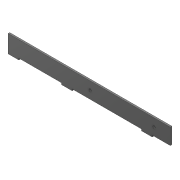
# Autodesk Inventor part: Divisória-30cm c rolamento
Saved by Autodesk Inventor 2020 (Build 240168000, 168)
## iProperties
Created: 2021-09-21
Part Number: Divisória-30cm c rolamento
Material: Generic
Document SubType Name: Modeling
Designer: pablo
Density: 1 g/cm^3
Appearance: Smooth - Black
Author: pablo
Autodesk Inventor part; units mm, degrees
ref_plane "YZ Plane" through (0, 0, 0) normal (1, 0, 0) x (0, 1, 0)
ref_plane "XZ Plane" through (0, 0, 0) normal (0, 1, 0) x (-1, 0, 0)
ref_plane "XY Plane" through (0, 0, 0) normal (0, 0, 1) x (1, 0, 0)
sketch "Sketch1" plane through (0, 0, 0) normal (0, 0, 1) x (1, 0, 0)
  line L0 (-152, 15) -> (152, 15)
  line L1 (152, 15) -> (152, -15)
  line L2 (152, -15) -> (-152, -15)
  line L3 (-152, -15) -> (-152, 15)
  line L4 (-152, 15) -> (152, -15) construction
  line L5 (152, 15) -> (-152, -15) construction
  point P0 (0, 0)
  dimension "d0" = 304
  dimension "d1" = 30
  constraints: 12 end point, 2 midpoint, 2 parallel, 1 horizontal, 1 perpendicular
  measures "d0" distance of L1.end L2.end
  measures "d1" distance of L0.end L1.end
extrude "Base" add sketch "Sketch1" along normal blind 3
sketch "Sketch2" plane through (0, 0, 3) normal (0, 0, 1) x (1, 0, 0)
  line L0 (-152, -15) -> (152, -15) projected
  line L1 (-152, -15) -> (-132, -15)
  line L2 (-132, -15) -> (-132, -18)
  line L3 (-132, -18) -> (-152, -18)
  line L4 (-152, -18) -> (-152, -15)
  line L5 (-102, -15) -> (-82, -15)
  line L6 (-82, -15) -> (-82, -18)
  line L7 (-82, -18) -> (-102, -18)
  line L8 (-102, -18) -> (-102, -15)
  line L9 (-52, -15) -> (-32, -15)
  line L10 (-32, -15) -> (-32, -18)
  line L11 (-32, -18) -> (-52, -18)
  line L12 (-52, -18) -> (-52, -15)
  line L13 (-2, -15) -> (18, -15)
  line L14 (18, -15) -> (18, -18)
  line L15 (18, -18) -> (-2, -18)
  line L16 (-2, -18) -> (-2, -15)
  line L17 (48, -15) -> (68, -15)
  line L18 (68, -15) -> (68, -18)
  line L19 (68, -18) -> (48, -18)
  line L20 (48, -18) -> (48, -15)
  line L21 (98, -15) -> (118, -15)
  line L22 (118, -15) -> (118, -18)
  line L23 (118, -18) -> (98, -18)
  line L24 (98, -18) -> (98, -15)
  point P0 (0, 0)
  point P1 (18, -15)
  point P2 (-2, -15)
  point P3 (-32, -15)
  point P4 (-132, -15)
  point P5 (68, -15)
  point P6 (48, -15)
  point P7 (-82, -15)
  point P8 (-102, -15)
  point P9 (118, -15)
  point P10 (98, -15)
  dimension "d4" = 20
  dimension "d5" = 3
  dimension "d8" = 50
  dimension "d21" = 34
  constraints: 48 end point, 2 horizontal, 2 parallel, 1 perpendicular, 40 other
  measures "d4" distance of L2.end L3.end
  measures "d5" distance of L1.end L2.end
  measures "d8" distance of L2.end L6.end
  measures "d21" horizontal distance of L22.end L0.end
extrude "Encaixe" add sketch "Sketch2" against normal blind 3 contours L0 L2 L3 L4 | L0 L10 L11 L12 | L0 L22 L23 L24
sketch "Sketch3" plane through (0, 0, 3) normal (0, 0, 1) x (1, 0, 0)
  circle A0 centre (122, 0) radius 2.5
  circle A1 centre (2, 0) radius 2.5
  line L0 (152, -15) -> (152, 15) projected
  dimension "d16" = 5
  dimension "d17" = 5
  dimension "d20" = 30
  dimension "d22" = 120
  constraints: 2 centre point, 1 coincident
  measures "d16" diameter of A0
  measures "d17" diameter of A1
  measures "d20" distance from line of L0 A0.centre
  measures "d22" distance of point (2, 0) A0.centre
extrude "Extrusion3" cut sketch "Sketch3" against normal blind 10
body "Solid1"
